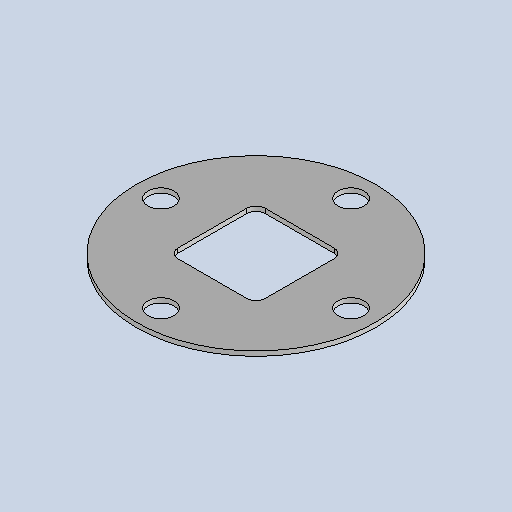
# Autodesk Inventor part: TZS 1757 FDS 940x50 FLANGE
Saved by Autodesk Inventor 2025.1 (Build 291241020, 241B)
## iProperties
Created: 2025-06-24
Part Number: TZS 1757 FDS 940x50 FLANGE
Material: Stainless Steel
Description: DIE16(5)|\ 90°|corrY -___°|X_____|bom___
Document SubType Name: Sheet Metal
Designer: user
Mass: 359.698 g
Surface Area: 327.391 cm^2
Volume: 44.9623 cm^3
Density: 8 g/cm^3
Flat Pattern Width: 15.6 cm
Flat Pattern Length: 15.6 cm
Flat Pattern Area: 243.36 cm^2
Sheet Metal Rule: Default
Sheet Metal Width: 156.000 mm
Sheet Metal Length: 156.000 mm
Sheet Metal Area: 24336.000 mm^2
Appearance: Default
Author: user
Autodesk Inventor part; units mm, degrees
ref_plane "YZ Plane" through (0, 0, 0) normal (1, 0, 0) x (0, 1, 0)
ref_plane "XZ Plane" through (0, 0, 0) normal (0, 1, 0) x (-1, 0, 0)
ref_plane "XY Plane" through (0, 0, 0) normal (0, 0, 1) x (1, 0, 0)
sketch "Sketch1" plane through (0, 0, 0) normal (0, 0, 1) x (1, 0, 0)
  circle A0 centre (0, 0) radius 78
  line L0 (28.5, 28.5) -> (-28.5, 28.5)
  line L1 (-28.5, 28.5) -> (-28.5, -28.5)
  line L2 (-28.5, -28.5) -> (28.5, -28.5)
  line L3 (28.5, -28.5) -> (28.5, 28.5)
  line L4 (28.5, 28.5) -> (-28.5, -28.5) construction
  line L5 (-28.5, 28.5) -> (28.5, -28.5) construction
  dimension "d157" = 156
  dimension "d158" = 57
  dimension "d159" = 57
  measures "d157" diameter of A0
  measures "d158" distance of L2.end L1.end
  measures "d159" distance of L1.end L0.end
extrude "Plate5" add sketch "Sketch1" along normal blind 3
sketch "Sketch7" plane through (0, 0, 0) normal (0, 0, -1) x (-1, 0, 0)
  circle A0 centre (0, 62) radius 8.5
  point P0 (0, 0)
  dimension "d160" = 17
  dimension "d161" = 62
  constraints: 1 centre point, 1 vertical alignment
  measures "d160" diameter of A0
  measures "d161" distance of point (0, 0) A0.centre
extrude "Cut1" cut sketch "Sketch7" against normal blind 3
pattern_circular "Circular Pattern1" count 4 over 360 about axis through (0, 0, -10) along (0, 0, 1) of "Cut1"
fillet "Corner Round1" radius 6 4 edges at (-28.5, -28.5, 1.5) (28.5, -28.5, 1.5) (28.5, 28.5, 1.5) (-28.5, 28.5, 1.5)
body "Solid3"
